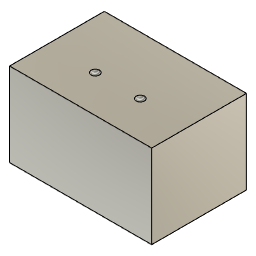
light_gate_holder v5 (Autodesk Fusion 360 design; units mm, degrees)
Autodesk Fusion 360 part; units mm, degrees
note: some values were not read from the file. Chosen so that the rebuilt part matches the saved one: which face or edge a step refers to; how an offset face is resized.
sketch "Sketch1" plane through (0, 0, 0) normal (0, 0, 1) x (1, 0, 0)
  line L0 (0, 0) -> (60, 0)
  line L1 (60, 0) -> (60, 60)
  line L2 (60, 60) -> (0, 60)
  line L3 (0, 60) -> (0, 0)
  dimension "d1" = 60
  dimension "d2" = 60
  constraint horizontal L0
  constraint vertical L1
  constraint horizontal L2
  constraint vertical L3
  constraint coincident L0.start L3.end
  measures "d1" distance of L0.start L0.end
  measures "d2" distance of L0.start L2.end
extrude "Extrude1" add sketch "Sketch1" along normal blind 10
sketch "Sketch2" plane through (0, 0, 10) normal (0, 0, 1) x (-1, 0, 0)
  line L0 (0, -60) -> (0, 0)
  line L1 (0, 0) -> (-60, 0)
  line L2 (-60, 0) -> (-60, -60)
  line L3 (-60, -60) -> (0, -60)
  line L4 (0, -60) -> (-30, -60)
  line L5 (-30, -60) -> (-30, -30)
  line L6 (-30, -30) -> (0, -30)
  line L7 (0, -30) -> (0, -60)
  dimension "d5" = 30
  constraint horizontal L4
  constraint vertical L5
  constraint horizontal L6
  constraint vertical L7
  constraint coincident L0.start L3.end
  measures "d5" distance of L0.start L6.end
sketch "Sketch3" plane through (0, 0, 10) normal (0, 0, 1) x (-1, 0, 0)
  line L0 (-30, -60) -> (-10, -60)
  line L1 (-10, -60) -> (-10, -30)
  line L2 (-10, -30) -> (-30, -30)
  line L3 (-30, -30) -> (-30, -60)
  line L4 (-30, -60) -> (-50, -60)
  line L5 (-50, -60) -> (-50, -30)
  line L6 (-50, -30) -> (-30, -30)
  line L7 (-30, -30) -> (-30, -60)
  dimension "d6" = 30
  dimension "d7" = 20
  dimension "d8" = 30
  constraint horizontal L0
  constraint vertical L1
  constraint horizontal L2
  constraint vertical L3
  constraint horizontal L4
  constraint vertical L5
  constraint horizontal L6
  constraint vertical L7
  measures "d6" distance of L0.start L2.end
  measures "d7" distance of L0.start L4.end
  measures "d8" distance of L0.start L2.end
extrude "Extrude2" add sketch "Sketch3" along normal blind 3.3
extrude "Extrude3" add 1 faces at (36.6667, 40, 13.3) along direction (0, 0, 1) blind 1
sketch "Sketch4" plane through (0, 0, 10) normal (0, 0, 1) x (-1, 0, 0)
  line L0 (0, -60) -> (-10, -60)
  line L1 (-10, -60) -> (-10, 0)
  line L2 (-10, 0) -> (0, 0)
  line L3 (0, 0) -> (0, -60)
  line L4 (-60, -60) -> (-50, -60)
  line L5 (-50, -60) -> (-50, 0)
  line L6 (-50, 0) -> (-60, 0)
  line L7 (-60, 0) -> (-60, -60)
  dimension "d25" = 10
  dimension "d26" = 60
  dimension "d27" = 10
  dimension "d28" = 60
  constraint horizontal L0
  constraint vertical L1
  constraint horizontal L2
  constraint vertical L3
  constraint horizontal L4
  constraint vertical L5
  constraint horizontal L6
  constraint vertical L7
  measures "d25" distance of L0.start L0.end
  measures "d26" distance of L0.start L2.end
  measures "d27" distance of L4.start L4.end
  measures "d28" distance of L4.start L6.end
extrude "Extrude4" cut sketch "Sketch4" against normal blind 5
sketch "Sketch5" plane through (0, 0, 10) normal (0, 0, 1) x (-1, 0, 0)
  circle A0 centre (-30, -15) radius 5
  dimension "d31" = 10
  measures "d31" diameter of A0
extrude "Extrude5" cut sketch "Sketch5" against normal blind 14
extrude "Extrude6" cut 1 faces at (15, 15, 10) along direction (0, 0, -1) blind 5
extrude "Extrude7" cut 1 faces at (40, 0, 3.3333) along direction (0, 1, 0) blind 2.021
extrude "Extrude8" cut 1 faces at (11.6667, 15.6737, 5) along direction (0, 0, -1) blind 3
sketch "Sketch6" plane through (0, 0, 2) normal (0, 0, 1) x (-1, 0, 0)
  line L0 (0, -2.021) -> (-60, -2.021)
  line L1 (-60, -2.021) -> (-60, -60)
  line L2 (-60, -60) -> (-50, -60)
  line L3 (-50, -60) -> (-50, -30)
  line L4 (-50, -30) -> (-10, -30)
  line L5 (-10, -30) -> (-10, -60)
  line L6 (-10, -60) -> (0, -60)
  line L7 (0, -60) -> (0, -2.021)
  circle A0 centre (-30, -15) radius 5
  line L8 (0, -2.021) -> (-5, -2.021)
  line L9 (-5, -2.021) -> (-5, -32.021)
  dimension "d40" = 30
  constraint coincident L0.start L7.end
  constraint coincident L0 L8.end
  constraint perpendicular L0 L9
  measures "d40" distance of L8.end L9.end
hole "Hole1" at (5, 32.021, 2) direction (0, 0, -1) diameter 3.529 depth 5 tip angle 118
thread "Thread1" "ISO Metric profile 4.0 M4x0.5 6H"
sketch "Sketch7" plane through (0, 0, 2) normal (0, 0, 1) x (-1, 0, 0)
  circle A0 centre (-5, -32.021) radius 1.7644
  line L0 (0, -2.021) -> (-60, -2.021)
  line L1 (-60, -2.021) -> (-60, -60)
  line L2 (-60, -60) -> (-50, -60)
  line L3 (-50, -60) -> (-50, -30)
  line L4 (-50, -30) -> (-10, -30)
  line L5 (-10, -30) -> (-10, -60)
  line L6 (-10, -60) -> (0, -60)
  line L7 (0, -60) -> (0, -2.021)
  circle A1 centre (-30, -15) radius 5
  line L8 (-60, -2.021) -> (-55, -2.021)
  line L9 (-55, -2.021) -> (-55, -32.021)
  dimension "d44" = 5
  dimension "d45" = 30
  constraint coincident L0.end L1.start
  constraint perpendicular L1 L8
  constraint perpendicular L0 L9
  measures "d44" distance of L0.end L8.end
  measures "d45" distance of L8.end L9.end
hole "Hole2" at (55, 32.021, 2) direction (0, 0, -1) diameter 3.529 depth 5 tip angle 118
thread "Thread2" "ISO Metric profile 4.0 M4x0.5 6H"
delete_face "DeleteFace1" 1 faces at (55.1757, 30.2653, 1.3333)
delete_face "DeleteFace2" 1 faces at (5.1757, 30.2653, 1.3333)
sketch "Sketch8" plane through (0, 0, 14.3) normal (0, 0, 1) x (-1, 0, 0)
  line L0 (-50, -60) -> (-10, -60)
  line L1 (-10, -60) -> (-10, -30)
  line L2 (-10, -30) -> (-50, -30)
  line L3 (-50, -30) -> (-50, -60)
  line L4 (-10, -30) -> (-20.5, -30)
  line L5 (-20.5, -30) -> (-20.5, -44.3)
  line L6 (-20.5, -44.3) -> (-10, -44.3)
  line L7 (-10, -44.3) -> (-10, -30)
  line L8 (-50, -30) -> (-39.5, -30)
  line L9 (-39.5, -30) -> (-39.5, -44.3)
  line L10 (-39.5, -44.3) -> (-50, -44.3)
  line L11 (-50, -44.3) -> (-50, -30)
  dimension "d49" = 10.5
  dimension "d50" = 14.3
  dimension "d51" = 10.5
  dimension "d52" = 14.3
  constraint horizontal L4
  constraint vertical L5
  constraint horizontal L6
  constraint vertical L7
  constraint coincident L1.end L2.start
  constraint horizontal L8
  constraint vertical L9
  constraint horizontal L10
  constraint vertical L11
  constraint coincident L2.end L3.start
  measures "d49" distance of L1.end L4.end
  measures "d50" distance of L1.end L6.end
  measures "d51" distance of L2.end L8.end
  measures "d52" distance of L2.end L10.end
hole "Hole3" at (20.5, 44.3, 14.3) at (39.5, 44.3, 14.3) direction (0, 0, -1) diameter 3.332 depth 10 tip angle 180
thread "Thread3" "ISO Metric profile 4.0 M4x0.5 6H" major diameter 4.0861 minor diameter 3.5287 pitch 0.5 angle 60 resizes the face on face at (20.583, 42.6361, 10.9667) on face at (38.7032, 45.7631, 10.9667)
extrude "Extrude9" cut 1 faces at (27.0885, 55.2965, 14.3) along direction (0, 0, -1) blind 12.3
extrude "Extrude10" cut 2 faces at (39.4715, 43.8368, 4.3) (20.4715, 43.8368, 4.3) along direction (0, 0, -1) blind 2.3
extrude "Extrude11" add 1 faces at (20, 2.021, 0.6667) along direction (0, -1, 0) blind 2.021
delete_face "DeleteFace3" 1 faces at (25.0248, 15.4978, 1.3333)
sketch "Sketch9" plane through (0, 0, 2) normal (0, 0, 1) x (-1, 0, 0)
  line L0 (-60, 0) -> (-60, -60)
  line L1 (-60, -60) -> (0, -60)
  line L2 (0, -60) -> (0, 0)
  line L3 (0, 0) -> (-60, 0)
  line L4 (-30, 0) -> (-30, -10)
  circle A0 centre (-30, -10) radius 5
  dimension "d66" = 10
  dimension "d67" = 10
  constraint midpoint L3 L4.start
  constraint perpendicular L3 L4
  constraint coincident L4.end A0.centre
  measures "d66" distance of L4.start L4.end
  measures "d67" diameter of A0
extrude "Extrude12" cut sketch "Sketch9" against normal blind 4 contours A0
sketch "Sketch10" plane through (0, 0, 0) normal (0, 0, -1) x (1, 0, 0)
  circle A0 centre (30, -10) radius 5
  line L0 (0, 0) -> (0, -60)
  line L1 (0, -60) -> (60, -60)
  line L2 (60, -60) -> (60, 0)
  line L3 (60, 0) -> (0, 0)
  line L4 (0, -60) -> (20, -60)
  line L5 (20, -60) -> (20, -55)
  line L6 (20, -55) -> (0, -55)
  line L7 (0, -55) -> (0, -60)
  line L8 (60, -60) -> (40, -60)
  line L9 (40, -60) -> (40, -55)
  line L10 (40, -55) -> (60, -55)
  line L11 (60, -55) -> (60, -60)
  dimension "d74" = 20
  dimension "d75" = 5
  dimension "d76" = 20
  dimension "d77" = 5
  constraint horizontal L4
  constraint vertical L5
  constraint horizontal L6
  constraint vertical L7
  constraint coincident L0 L1.start
  constraint horizontal L8
  constraint vertical L9
  constraint horizontal L10
  constraint vertical L11
  constraint coincident L1.end L2.start
  measures "d74" distance of L0.end L4.end
  measures "d75" distance of L0.end L6.end
  measures "d76" distance of L1.end L8.end
  measures "d77" distance of L1.end L10.end
hole "Hole4" at (20, 55, 0) at (40, 55, 0) direction (0, 0, 1) diameter 4.5 depth 5 tip angle 180
sketch "Sketch11" plane through (0, 0, 0) normal (0, 0, -1) x (1, 0, 0)
  circle A0 centre (20, -55) radius 2.25
  circle A1 centre (40, -55) radius 2.25
  circle A2 centre (30, -10) radius 5
  line L0 (0, 0) -> (0, -60)
  line L1 (0, -60) -> (60, -60)
  line L2 (60, -60) -> (60, 0)
  line L3 (60, 0) -> (0, 0)
  line L4 (20, -55) -> (30, -55)
  line L5 (30, -55) -> (30, -35)
  line L6 (30, -35) -> (20, -35)
  line L7 (20, -35) -> (20, -55)
  dimension "d81" = 10
  dimension "d82" = 20
  constraint horizontal L4
  constraint vertical L5
  constraint horizontal L6
  constraint vertical L7
  constraint coincident A0.centre L4.start
  measures "d81" distance of A0.centre L4.end
  measures "d82" distance of A0.centre L6.end
hole "Hole5" at (30, 35, 0) direction (0, 0, 1) diameter 4.5 depth 5 tip angle 180
sketch "Sketch12" plane through (0, 0, 2) normal (0, 0, 1) x (-1, 0, 0)
  circle A0 centre (-30, -35) radius 2.25
  circle A1 centre (-20, -55) radius 2.25
  circle A2 centre (-40, -55) radius 2.25
  circle A3 centre (-30, -10) radius 5
  line L0 (-60, 0) -> (-60, -60)
  line L1 (-60, -60) -> (0, -60)
  line L2 (0, -60) -> (0, 0)
  line L3 (0, 0) -> (-60, 0)
  line L4 (0, 0) -> (-5, 0)
  line L5 (-5, 0) -> (-5, -30)
  line L6 (-5, -30) -> (0, -30)
  line L7 (0, -30) -> (0, 0)
  line L8 (-60, 0) -> (-55, 0)
  line L9 (-55, 0) -> (-55, -30)
  line L10 (-55, -30) -> (-60, -30)
  line L11 (-60, -30) -> (-60, 0)
  dimension "d90" = 5
  dimension "d91" = 30
  dimension "d92" = 5
  dimension "d93" = 30
  constraint horizontal L4
  constraint vertical L5
  constraint horizontal L6
  constraint vertical L7
  constraint coincident L2.end L3.start
  constraint horizontal L8
  constraint vertical L9
  constraint horizontal L10
  constraint vertical L11
  constraint coincident L0.start L3.end
  measures "d90" distance of L2.end L4.end
  measures "d91" distance of L2.end L6.end
  measures "d92" distance of L0.start L8.end
  measures "d93" distance of L0.start L10.end
hole "Hole6" at (5, 30, 2) at (55, 30, 2) direction (0, 0, -1) diameter 4.5 depth 30 tip angle 180
delete_face "DeleteFace4" 1 faces at (25.0062, 10.2492, 0.6667)
delete_face "DeleteFace5" 1 faces at (5.224, 27.7612, 1.3333)
delete_face "DeleteFace6" 1 faces at (27.8672, 35.7166, 0.6667)
delete_face "DeleteFace7" 1 faces at (55.224, 32.2388, 1.3333)
delete_face "DeleteFace8" 1 faces at (38.313, 56.4888, 0.6667)
delete_face "DeleteFace9" 1 faces at (17.8672, 55.7166, 0.6667)
extrude "Extrude13" add 1 faces at (20, 40, 2) along direction (0, 0, 1) blind 33.308
extrude "Extrude14" cut 1 faces at (40, 60, 23.5387) along direction (0, -1, 0) blind 20
sketch "Sketch13" plane through (0, 0, 0) normal (0, 0, -1) x (1, 0, 0)
  line L0 (0, -40) -> (60, -40)
  line L1 (60, -40) -> (60, 0)
  line L2 (60, 0) -> (0, 0)
  line L3 (0, 0) -> (0, -40)
  line L4 (0, -40) -> (5, -40)
  line L5 (5, -40) -> (5, -35)
  line L6 (5, -35) -> (0, -35)
  line L7 (0, -35) -> (0, -40)
  line L8 (5, -35) -> (55, -35)
  line L9 (55, -35) -> (55, -5)
  line L10 (55, -5) -> (5, -5)
  line L11 (5, -5) -> (5, -35)
  dimension "d101" = 5
  dimension "d102" = 5
  dimension "d103" = 50
  dimension "d104" = 30
  constraint horizontal L4
  constraint vertical L5
  constraint horizontal L6
  constraint vertical L7
  constraint coincident L0.start L3.end
  constraint horizontal L8
  constraint vertical L9
  constraint horizontal L10
  constraint vertical L11
  measures "d101" distance of L0.start L4.end
  measures "d102" distance of L0.start L6.end
  measures "d103" distance of L5.end L8.end
  measures "d104" distance of L5.end L10.end
hole "Hole7" at (5, 5, 0) at (55, 5, 0) at (5, 35, 0) at (55, 35, 0) direction (0, 0, 1) diameter 6.78 depth 20 tip angle 180
thread "Thread4" "ISO Metric profile 8.0 M8x1 6H" major diameter 8.147 minor diameter 7.035 pitch 1 angle 60 resizes the face on face at (5.169, 8.3858, 6.6667) on face at (55.169, 8.3858, 6.6667) on face at (5.169, 38.3858, 6.6667) on face at (55.169, 38.3858, 6.6667)
sketch "Sketch14" plane through (0, 0, 35.308) normal (0, 0, 1) x (-1, 0, 0)
  line L0 (-60, -40) -> (0, -40)
  line L1 (0, -40) -> (0, 0)
  line L2 (0, 0) -> (-60, 0)
  line L3 (-60, 0) -> (-60, -40)
  line L4 (0, 0) -> (-30, 0)
  line L5 (-30, 0) -> (-30, -15.7)
  line L6 (-30, -15.7) -> (0, -15.7)
  line L7 (0, -15.7) -> (0, 0)
  line L8 (-30, -15.7) -> (-39.5, -15.7)
  line L9 (-30, -15.7) -> (-20.5, -15.7)
  dimension "d108" = 30
  dimension "d109" = 15.7
  dimension "d110" = 9.5
  dimension "d111" = 9.5
  constraint horizontal L4
  constraint vertical L5
  constraint horizontal L6
  constraint vertical L7
  constraint coincident L1.end L2.start
  constraint perpendicular L5 L8
  constraint perpendicular L5 L9
  measures "d108" distance of L1.end L4.end
  measures "d109" distance of L1.end L6.end
  measures "d110" distance of L5.end L8.end
  measures "d111" distance of L5.end L9.end
hole "Hole8" at (20.5, 15.7, 35.308) at (39.5, 15.7, 35.308) direction (0, 0, -1) diameter 3.332 depth 10 tip angle 180
thread "Thread5" "ISO Metric profile 4.0 M4x0.5 6H" major diameter 4.0861 minor diameter 3.5287 pitch 0.5 angle 60 resizes the face on face at (19.4291, 16.9762, 31.9747) on face at (38.9302, 17.2655, 31.9747)
equation "d110 = ( 19 / 2 ) * 1 mm"
equation "d111 = ( 19 / 2 ) * 1 mm"
